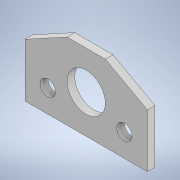
# Autodesk Inventor part: Assignment 1.3 - Positioning Stop
Saved by Autodesk Inventor 2021.1 (Build 251245000, 245)
## iProperties
Created: 2021-05-12
Part Number: Assignment 1.3 - Positioning Stop
Material: Generic
Document SubType Name: Modeling
Designer: as000166
Density: 1 g/cm^3
Appearance: Default
Author: as000166
Autodesk Inventor part; units mm, degrees
ref_plane "YZ Plane" through (0, 0, 0) normal (1, 0, 0) x (0, 1, 0)
ref_plane "XZ Plane" through (0, 0, 0) normal (0, 1, 0) x (-1, 0, 0)
ref_plane "XY Plane" through (0, 0, 0) normal (0, 0, 1) x (1, 0, 0)
sketch "Sketch1" plane through (0, 0, 0) normal (0, 0, 1) x (1, 0, 0)
  line L0 (101.6, 0) -> (101.6, 44.45)
  line L1 (0, 0) -> (0, 44.45)
  line L2 (50.8, 63.5) -> (66.675, 63.5)
  line L3 (50.8, 63.5) -> (34.925, 63.5)
  line L4 (0, 44.45) -> (34.925, 63.5)
  line L5 (66.675, 63.5) -> (101.6, 44.45)
  circle A0 centre (50.8, 31.75) radius 15.875
  circle A1 centre (19.05, 19.05) radius 6.35
  circle A2 centre (82.55, 19.05) radius 6.35
  line L6 (0, 0) -> (101.6, 0)
  dimension "d1" = 44.45
  dimension "d3" = 44.45
  dimension "d5" = 15.875
  dimension "d6" = 15.875
  dimension "d8" = 31.75
  dimension "d11" = 12.7
  dimension "d14" = 12.7
  dimension "d15" = 101.6
  constraints: 14 end point, 3 centre point, 3 horizontal, 1 vertical
  measures "d1" distance of L0.start L0.end
  measures "d3" distance of L1.start L1.end
  measures "d5" distance of L2.start L2.end
  measures "d6" distance of L2.start L3.end
  measures "d8" diameter of A0
  measures "d11" diameter of A1
  measures "d14" diameter of A2
  measures "d15" distance of L1.start L0.start
extrude "Extrusion1" add sketch "Sketch1" along normal blind 6.35
body "Solid1"
